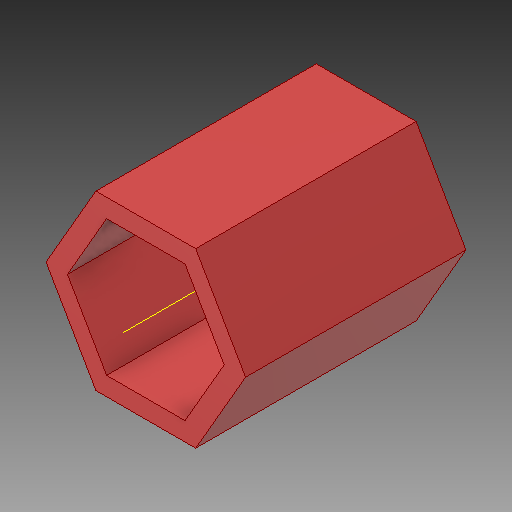
# Autodesk Inventor part: 1-2 TO 3-8 ADAPTER
Saved by Autodesk Inventor 2019.4 (Build 234330000, 330)
## iProperties
Created: 2020-01-26
Part Number: 1-2 TO 3-8 ADAPTER
Material: ABS Plastic
Document SubType Name: Modeling
Designer: mavericks
Density: 1.06 g/cm^3
Appearance: Smooth - Red
Author: mavericks
Autodesk Inventor part; units mm, degrees
ref_plane "YZ Plane" through (0, 0, 0) normal (1, 0, 0) x (0, 1, 0)
ref_plane "XZ Plane" through (0, 0, 0) normal (0, 1, 0) x (-1, 0, 0)
ref_plane "XY Plane" through (0, 0, 0) normal (0, 0, 1) x (1, 0, 0)
sketch "Sketch1" plane through (0, 0, 0) normal (0, 0, 1) x (1, 0, 0)
  line L0 (3.5929, 6.223) -> (7.1857, 0)
  line L1 (7.1857, 0) -> (3.5929, -6.223)
  line L2 (3.5929, -6.223) -> (-3.5929, -6.223)
  line L3 (-3.5929, -6.223) -> (-7.1857, 0)
  line L4 (-7.1857, 0) -> (-3.5929, 6.223)
  line L5 (-3.5929, 6.223) -> (3.5929, 6.223)
  line L6 (2.823, 4.8895) -> (5.6459, 0)
  line L7 (5.6459, 0) -> (2.823, -4.8895)
  line L8 (2.823, -4.8895) -> (-2.823, -4.8895)
  line L9 (-2.823, -4.8895) -> (-5.6459, 0)
  line L10 (-5.6459, 0) -> (-2.823, 4.8895)
  line L11 (-2.823, 4.8895) -> (2.823, 4.8895)
  point P0 (0, 0)
  point P1 (0, 0)
  point P2 (0, 0)
  dimension "d0" = 12.446
  dimension "d1" = 9.779
  constraints: 24 end point, 2 coincident, 2 horizontal, 26 other
  measures "d0" distance between parallel lines of L2 L5
  measures "d1" distance between parallel lines of L8 L11
extrude "Extrusion1" add sketch "Sketch1" along normal mid plane 15.875
body "Solid1"
